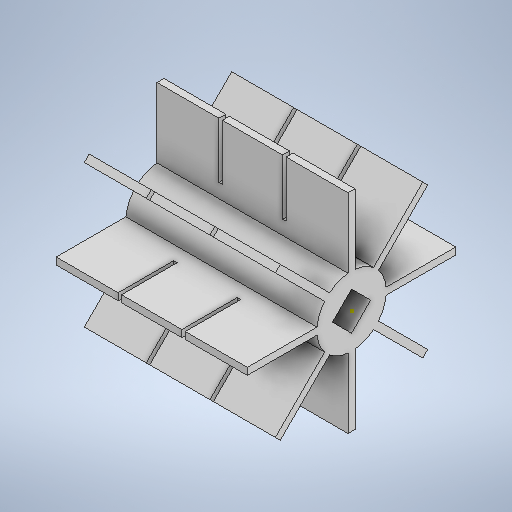
# Autodesk Inventor part: Hélice
Saved by Autodesk Inventor 2026.2 (Build 302298010, 298A)
## iProperties
Created: 2026-04-02
Part Number: Hélice
Material: Générique
Document SubType Name: Modeling
Designer: Genon
Density: 1 g/cm^3
Appearance: Par défaut
Author: Genon
Autodesk Inventor part; units mm, degrees
ref_plane "YZ Plane" through (0, 0, 0) normal (1, 0, 0) x (0, 1, 0)
ref_plane "XZ Plane" through (0, 0, 0) normal (0, 1, 0) x (-1, 0, 0)
ref_plane "XY Plane" through (0, 0, 0) normal (0, 0, 1) x (1, 0, 0)
sketch "Esquisse1" plane through (0, 0, 0) normal (0, 0, 1) x (1, 0, 0)
  line L0 (0, 0) -> (0, 10)
  line L1 (0, 10) -> (55, 10)
  line L2 (55, 10) -> (55, 0)
  line L3 (55, 0) -> (0, 0)
  line L4 (-11, 0) -> (66, 0) projected
  dimension "d0" = 10
  dimension "d1" = 55
  constraints: 8 end point, 2 perpendicular, 1 horizontal, 1 vertical
  measures "d0" distance of L0.start L0.end
  measures "d1" distance of L0.end L1.end
revolve "Révolution1" add sketch "Esquisse1" angle 360 about axis through (-10, 0, 0) along (1, 0, 0)
sketch "Esquisse2" plane through (55, 0, 0) normal (1, 0, 0) x (0, 0, -1)
  point P0 (0, 0)
sketch "Esquisse3" plane through (55, 0, 0) normal (1, 0, 0) x (0, 0, -1)
  circle A0 centre (0, 0) radius 10 projected
  line L0 (0, 10) -> (0, 30)
  line L1 (0, 30) -> (1, 30)
  line L2 (1, 30) -> (1, 9.9499)
  line L3 (0, 30) -> (-1, 30)
  line L4 (-1, 30) -> (-1, 9.9499)
  dimension "d4" = 20
  dimension "d5" = 1
  dimension "d6" = 1
  constraints: 10 end point, 3 perpendicular, 3 point on circle, 1 point on line, 1 vertical
  measures "d4" distance of L0.start L0.end
  measures "d5" distance of L0.end L1.end
  measures "d6" distance of L0.end L3.end
extrude "Extrusion1" add sketch "Esquisse3" against normal up to surface (55 mm away) contours A0 L0 L1 L2 | L4 L3 L0 A0
sketch "Esquisse4" plane through (55, 9.9499, 1) normal (0, 0, 1) x (1, 0, 0)
  line L0 (-55, 20.0501) -> (-55, 0) projected
  line L1 (-55, 20.0501) -> (-36.67, 20.0501)
  line L2 (0, 20.0501) -> (-55, 20.0501) projected
  line L3 (-36.67, 20.0501) -> (-18.34, 20.0501)
  line L4 (0, 20.0501) -> (0, 0) projected
  line L5 (-18.34, 20.0501) -> (0, 20.0501)
  line L6 (-36.67, 20.0501) -> (-36.67, 4.0501)
  line L7 (-36.67, 4.0501) -> (-36.17, 4.0501)
  line L8 (-36.17, 4.0501) -> (-36.17, 20.0501)
  line L9 (-36.67, 4.0501) -> (-37.17, 4.0501)
  line L10 (-37.17, 4.0501) -> (-37.17, 20.0501)
  line L11 (-18.34, 20.0501) -> (-18.34, 4.0501)
  line L12 (-18.34, 4.0501) -> (-18.84, 4.0501)
  line L13 (-18.84, 4.0501) -> (-18.84, 20.0501)
  line L14 (-18.34, 4.0501) -> (-17.84, 4.0501)
  line L15 (-17.84, 4.0501) -> (-17.84, 20.0501)
  point P0 (-55, -9.9499)
  dimension "d9" = 18.33
  dimension "d11" = 18.33
  dimension "d12" = 16
  dimension "d13" = 0.5
  dimension "d14" = 0.5
  dimension "d15" = 0.5
  dimension "d16" = 0.5
  constraints: 26 end point, 10 point on line, 6 perpendicular, 1 collinear, 1 parallel
  measures "d9" distance of L0.start L1.end
  measures "d11" distance of L1.end L3.end
  measures "d12" distance of L1.end L6.end
  measures "d13" distance of L6.end L7.end
  measures "d14" distance of L6.end L9.end
  measures "d15" distance of L11.end L12.end
  measures "d16" distance of L11.end L14.end
extrude "Extrusion2" cut sketch "Esquisse4" against normal through all
pattern_circular "Réseau circulaire1" count 8 over 360 about axis through (27.5, 0, 0) along (1, 0, 0) of "Extrusion2", "Extrusion1"
sketch "Esquisse5" plane through (0, 9.9499, 1) normal (-1, 0, 0) x (0, 0, 1)
  circle A0 centre (-1, -9.9499) radius 5.5
  line L0 (-1, -9.9499) -> (-1, -4.4499)
  line L1 (-1, -4.4499) -> (-6.5, -9.9499)
  line L2 (-6.5, -9.9499) -> (-1, -15.4499)
  line L3 (-1, -15.4499) -> (4.5, -9.9499)
  line L4 (4.5, -9.9499) -> (-1, -4.4499)
  dimension "d22" = 11
  constraints: 10 end point, 4 point on circle, 1 centre point, 1 coincident, 1 perpendicular, 1 point on line, 1 vertical
  measures "d22" diameter of A0
extrude "Extrusion3" cut sketch "Esquisse5" against normal through all contours L3 L2 L1 L4
